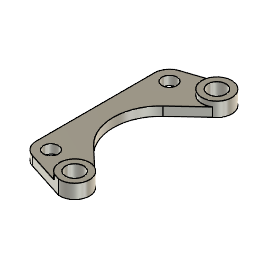
ex 2 (Autodesk Fusion 360 design; units mm, degrees)
part number: 2025-11-27-11-32-42-556
Autodesk Fusion 360 part; units mm, degrees
note: some values were not read from the file. Set by a fixed rule: which sketch regions a step uses.
sketch "Sketch1" plane through (0, 0, 0) normal (0, 0, 1) x (1, 0, 0)
  line L0 (0, 38.1) -> (0, -38.1)
  line L1 (-63.5, 0) -> (0, 0)
  circle A0 centre (0, 38.1) radius 4.826
  circle A1 centre (0, 38.1) radius 8.001
  circle A2 centre (-19.05, 31.75) radius 3.9751
  circle A3 centre (-19.05, 31.75) radius 8.001
  circle A4 centre (-19.05, -31.75) radius 3.9751
  circle A5 centre (-19.05, -31.75) radius 8.001
  circle A6 centre (0, -38.1) radius 4.826
  circle A7 centre (0, -38.1) radius 8.001
  circle A8 centre (8.001, 0) radius 25.4
  line L2 (4.3882, 31.4097) -> (-9.3568, 18.5436)
  line L3 (-27.051, 31.75) -> (-27.051, -31.75)
  line L4 (-21.5016, -39.3661) -> (-0.6654, -46.0733)
  line L5 (-2.5301, 45.6904) -> (-21.5801, 39.3404)
  line L6 (-9.5283, -18.3816) -> (3.7218, -31.0173)
  dimension "d1" = 76.2
  dimension "d2" = 9.652
  dimension "d3" = 16.002
  dimension "d4" = 7.9502
  dimension "d5" = 16.002
  dimension "d6" = 19.05
  dimension "d7" = 6.35
  dimension "d8" = 50.8
  constraint vertical L0
  constraint coincident L1.end origin
  constraint perpendicular L0 L1
  constraint coincident L0.start A0.centre
  constraint concentric A0 A1
  constraint concentric A2 A3
  constraint symmetric L1 A0 A6
  constraint symmetric L1 A1 A7
  constraint symmetric L1 A2 A4
  constraint symmetric L1 A3 A5
  constraint coincident A1 L2.start
  constraint coincident A8 L2.end
  constraint tangent A8 L2
  constraint coincident A3 L3.start
  constraint tangent A3 L3
  constraint coincident A5 L3.end
  constraint tangent A5 L3
  constraint coincident A5 L4.start
  constraint tangent A5 L4
  constraint coincident A7 L4.end
  constraint coincident A1 L5.start
  constraint tangent A1 L5
  constraint coincident A3 L5.end
  constraint tangent A3 L5
  constraint coincident A8 L6.start
  constraint tangent A8 L6
  constraint coincident A7 L6.end
  measures "d1" distance of L0.start L0.end
  measures "d2" diameter of A0
  measures "d3" diameter of A1
  measures "d4" diameter of A2
  measures "d5" diameter of A3
  measures "d6" horizontal distance of L0.start A2.centre
  measures "d7" vertical distance of L0.start A2.centre
  measures "d8" diameter of A8
extrude "Extrude1" add sketch "Sketch1" along normal blind 4.826 contours L0 A1 L2 | L0 L1 A1 A3 A8 L2 L3 L5 | A1 | A3 | L0 L1 A5 A7 A8 L3 L4 L6 | L0 A7 L6 | A5 | A7 L4 picked at (-2.134, -44.5605)
extrude "Extrude2" add sketch "Sketch1" along normal blind 7.62 contours A1 | A7 L4 picked at (-2.134, -44.5605)
